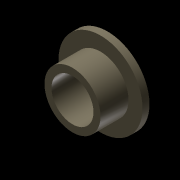
# Autodesk Inventor part: 80F-0605
Saved by Autodesk Inventor 2011 SP1 (Build 150282100, 282)
## iProperties
Created: 2013-02-08
Part Number: 80F-0605
Document SubType Name: Modeling
Designer: arihon
Density: 1 g/cm^3
Author: arihon
Autodesk Inventor part; units mm, degrees
ref_plane "YZ Plane" through (0, 0, 0) normal (1, 0, 0) x (0, 1, 0)
ref_plane "XZ Plane" through (0, 0, 0) normal (0, 1, 0) x (-1, 0, 0)
ref_plane "XY Plane" through (0, 0, 0) normal (0, 0, 1) x (1, 0, 0)
sketch "スケッチ1" plane through (0, 0, 0) normal (0, 0, 1) x (1, 0, 0)
  line L0 (0, 0) -> (0, 10)
  line L1 (-4, 6.5111) -> (-3, 6.5111)
  line L2 (-3, 6.5111) -> (-3, 1.5111)
  line L3 (-3, 1.5111) -> (-4, 1.5111)
  line L4 (-4, 1.5111) -> (-4, 6.5111)
  line L5 (-4, 6.5111) -> (-6, 6.5111)
  line L6 (-6, 6.5111) -> (-6, 5.5111)
  line L7 (-6, 5.5111) -> (-4, 5.5111)
  line L8 (-4, 5.5111) -> (-4, 6.5111)
  point P0 (0, 0)
  dimension "d0" = 10
  dimension "d1" = 6
  dimension "d2" = 0
  dimension "d3" = 1
  dimension "d4" = 1
  dimension "d5" = 12
  dimension "d6" = 5
  constraints: 18 end point, 4 parallel, 2 horizontal, 2 perpendicular, 1 vertical
  measures "d0" distance of L0.start L0.end
  measures "d1" diameter of L2 L0
  measures "d2" distance from line of point (0, 0) L0
  measures "d3" distance between parallel lines of L2 L4
  measures "d4" distance between parallel lines of L5 L7
  measures "d5" diameter of L6 L0
  measures "d6" distance of L1.end L2.end
revolve "回転1" add sketch "スケッチ1" angle 360 about axis through (0, 0, 0) along (0, 1, 0)
